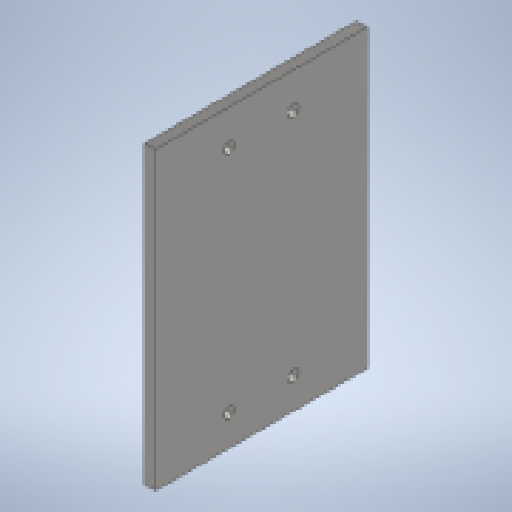
# Autodesk Inventor part: Z_Gantry_Plate
Saved by Autodesk Inventor 2023 (Build 270158000, 158)
## iProperties
Created: 2022-05-07
Part Number: Z_Gantry_Plate
Material: Steel, Mild
Document SubType Name: Modeling
Designer: plebbb
Density: 7.85 g/cm^3
Appearance: Semi-Polished
Mass: 1924.24 g
Surface Area: 706.63 cm^2
Volume: 245.125 cm^3
Author: plebbb
Autodesk Inventor part; units mm, degrees
ref_plane "YZ Plane" through (0, 0, 0) normal (1, 0, 0) x (0, 1, 0)
ref_plane "XZ Plane" through (0, 0, 0) normal (0, 1, 0) x (-1, 0, 0)
ref_plane "XY Plane" through (0, 0, 0) normal (0, 0, 1) x (1, 0, 0)
sketch "Sketch1" plane through (0, 0, 0) normal (1, 0, 0) x (0, 1, 0)
  line L0 (0, 0) -> (212.4, 0)
  line L1 (212.4, 0) -> (212.4, -152.4)
  line L2 (212.4, -152.4) -> (0, -152.4)
  line L3 (0, -152.4) -> (0, 0)
  dimension "d0" = 212.4
  dimension "d1" = 152.4
  constraints: 8 end point, 2 parallel, 1 horizontal, 1 perpendicular
  measures "d0" distance of L1.end L2.end
  measures "d1" distance of L0.end L1.end
extrude "Extrusion1" add sketch "Sketch1" along normal blind 7.62
sketch "Sketch2" plane through (7.62, 0, 0) normal (1, 0, 0) x (0, 0, -1)
  line L0 (53.2, 187) -> (99.2, 187) construction
  circle A0 centre (53.2, 187) radius 4
  circle A1 centre (99.2, 187) radius 4
  line L1 (0, 0) -> (152.4, 0) construction
  line L2 (53.2, 22.225) -> (99.2, 22.225) construction
  circle A2 centre (53.2, 22.225) radius 4
  circle A3 centre (99.2, 22.225) radius 4
  point P0 (76.2, 187)
  point P1 (76.2, 0)
  point P2 (76.2, 22.225)
  point P3 (76.2, 0)
  point P4 (76.2, 0)
  dimension "d4" = 8
  dimension "d5" = 187
  dimension "d6" = 46
  dimension "d9" = 8
  dimension "d10" = 46
  dimension "d11" = 22.225
  constraints: 5 midpoint, 4 centre point, 4 coincident, 4 end point, 2 equal radius, 2 horizontal, 2 vertical alignment
  measures "d4" diameter of A1
  measures "d5" distance from line of L1.start L0
  measures "d6" distance of L0.start L0.end
  measures "d9" diameter of A3
  measures "d10" distance of L2.start L2.end
  measures "d11" distance from line of point (76.2, 0) L2
extrude "Extrusion2" cut sketch "Sketch2" against normal blind 7.62
body "Solid1"
